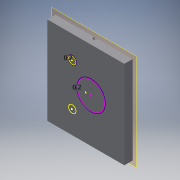
# Autodesk Inventor part: 00_PDMS_mould_1
Saved by Autodesk Inventor 2019.4 (Build 234330000, 330)
## iProperties
Created: 2021-04-19
Part Number: 00_PDMS_mould_1
Material: Generic
Document SubType Name: Modeling
Designer: diederichbenedict
Density: 1 g/cm^3
Appearance: Default
Author: diederichbenedict
Autodesk Inventor part; units mm, degrees
ref_plane "YZ Plane" through (0, 0, 0) normal (1, 0, 0) x (0, 1, 0)
ref_plane "XZ Plane" through (0, 0, 0) normal (0, 1, 0) x (-1, 0, 0)
ref_plane "XY Plane" through (0, 0, 0) normal (0, 0, 1) x (1, 0, 0)
ref_plane "Work Plane1" through (0, 0, 0) normal (0, 0, 1) x (1, 0, 0)
sketch "Sketch1" plane through (0, 0, 0) normal (0, 0, 1) x (1, 0, 0)
  arc A0 (2.9937, -6.1068) -> (2.9937, 6.1788) centre (1.841, 0.036) ccw projected
  line L0 (2.9937, -6.1068) -> (2.9937, -9.05) projected
  line L1 (2.9937, -9.05) -> (-5, -9.05) projected
  arc A1 (-5, -6.35) -> (-5, -9.05) centre (-5, -7.7) ccw projected
  line L2 (-5, -6.35) -> (-0.5216, -6.35) projected
  line L3 (-0.5216, -6.35) -> (-0.5216, -5.7502) projected
  arc A2 (-0.9246, 5.6409) -> (-0.5216, -5.7502) centre (1.841, 0.036) ccw projected
  line L4 (-0.9246, 5.6409) -> (-0.9246, 6.35) projected
  line L5 (-0.9246, 6.35) -> (-5, 6.35) projected
  arc A3 (-5, 9.05) -> (-5, 6.35) centre (-5, 7.7) ccw projected
  line L6 (-5, 9.05) -> (2.9937, 9.05) projected
  line L7 (2.9937, 9.05) -> (2.9937, 6.1788) projected
  line L8 (14, -16) -> (-14, -16) projected
  line L9 (14, 16) -> (14, -16) projected
  line L10 (-14, 16) -> (14, 16) projected
  line L11 (-14, -16) -> (-14, 16) projected
  point P0 (0, 0)
extrude "Extrusion1" add sketch "Sketch1" along normal blind 3 contours L0 L1 A1 L2 L3 A2 L4 L5 A3 L6 L7 A0 | L8 L11 L10 L9
sketch "Sketch2" plane through (0, 0, 3) normal (0, 0, 1) x (1, 0, 0)
  circle A0 centre (-5, 7.7) radius 1.35 projected
  circle A1 centre (-5, -7.7) radius 1.35 projected
  circle A2 centre (1.841, 0.036) radius 5 projected
  circle A3 centre (1.841, 0.036) radius 5.2
  circle A4 centre (-5, 7.7) radius 1.55
  point P0 (0, 0)
  dimension "d2" = 0.2
  dimension "d3" = 0.2
  constraints: 2 centre point
  measures "d2" radial gap between concentric circles of A2 A3
  measures "d3" radial gap between concentric circles of A0 A4
sketch "Sketch3" plane through (0, 0, 0) normal (0, 0, -1) x (-1, 0, 0)
  circle A0 centre (5, 7.7) radius 2.5 projected
  circle A1 centre (5, -7.7) radius 2.5 projected
  point P0 (0, 0)
extrude "Extrusion2" cut sketch "Sketch3" against normal through all
sketch "Sketch4" plane through (0, 0, 0) normal (0, 0, -1) x (-1, 0, 0)
  line L0 (-14, -16) -> (14, -16) projected
  line L1 (14, -16) -> (14, 16) projected
  line L2 (14, 16) -> (-14, 16) projected
  line L3 (-14, 16) -> (-14, -16) projected
  line L4 (9, -11.7) -> (9, 11.7) projected
  line L5 (-9, -11.7) -> (9, -11.7) projected
  line L6 (-9, 11.7) -> (-9, -11.7) projected
  line L7 (9, 11.7) -> (-9, 11.7) projected
  point P0 (0, 0)
extrude "Extrusion3" cut sketch "Sketch4" against normal blind 1 contours L5 L6 L7 L4
sketch "Sketch5" plane through (0, 0, 3) normal (0, 0, 1) x (1, 0, 0)
  circle A0 centre (-5, 7.7) radius 2.5 projected
  circle A1 centre (-5, -7.7) radius 2.5 projected
  point P0 (0, 0)
ref_plane "Work Plane2" through (-6.35, -9.05, 2.6) normal (0, 0, 1) x (1, 0, 0)
extrude "Extrusion4" add sketch "Sketch5" against normal up to surface (0.4 mm away)
sketch "Sketch6" plane through (-14, 16, 0) normal (0, 1, 0) x (1, 0, 0)
  line L0 (23, -1) -> (5, -1) projected
  line L1 (0, 0) -> (28, 0) projected
  line L2 (0, 0) -> (0, -3) projected
  line L3 (28, -3) -> (0, -3) projected
  line L4 (28, 0) -> (28, -3) projected
  circle A0 centre (14.7595, -0.2282) radius 0.75
  dimension "d11" = 1.5
  constraints: 1 centre point
  measures "d11" diameter of A0
extrude "Extrusion5" cut sketch "Sketch6" against normal through all contours A0 L1 | L1 A0
body "Solid1"
